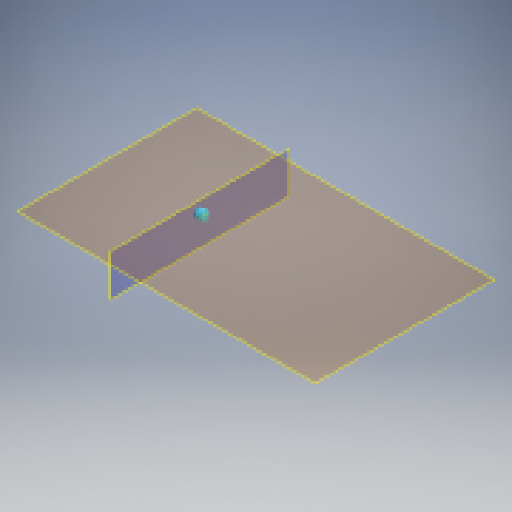
# Autodesk Inventor part: kicker
Saved by Autodesk Inventor 2023 (Build 270158000, 158)
## iProperties
Created: 2025-03-27
Part Number: kicker
Material: Типовые
Document SubType Name: Modeling
Designer: Ivan
Density: 1 g/cm^3
Appearance: Серо-синий
Author: Ivan
Autodesk Inventor part; units mm, degrees
ref_plane "YZ Plane" through (0, 0, 0) normal (1, 0, 0) x (0, 1, 0)
ref_plane "XZ Plane" through (0, 0, 0) normal (0, 1, 0) x (-1, 0, 0)
ref_plane "XY Plane" through (0, 0, 0) normal (0, 0, 1) x (1, 0, 0)
sketch "Эскиз1" plane through (0, 0, 0) normal (1, 0, 0) x (0, 1, 0)
  circle A0 centre (0, 0) radius 2.067 construction
  circle A1 centre (0, 0) radius 5
  circle A2 centre (0, 0) radius 6
  circle A3 centre (0, 0) radius 2.467 projected
  point P0 (0, 0)
  dimension "d1" = 10
  dimension "d2" = 12
  constraints: 2 centre point, 2 coincident
  measures "d1" diameter of A1
  measures "d2" diameter of A2
extrude "Выдавливание1" add sketch "Эскиз1" along normal blind 6.7 contours A2
sketch "Эскиз4" plane through (0, 0, 0) normal (-1, 0, 0) x (0, 0, 1)
  circle A0 centre (0, 0) radius 6 projected
  circle A1 centre (0, 0) radius 5 projected
  point P0 (0, 0)
extrude "Выдавливание2" add sketch "Эскиз4" along normal blind 2.64 contours A0 | A1
ref_plane "РабПлоскость1" through (0, 0, 0) normal (0, 1, 0) x (-1, 0, 0)
sketch "Эскиз5" plane through (0, 0, 0) normal (0, 1, 0) x (-1, 0, 0)
  line L0 (2.64, -6) -> (-6.7, -6) projected
  line L1 (-5, 6) -> (0, 6)
  line L2 (0, 6) -> (0, -6)
  line L3 (0, -6) -> (-5, -6)
  line L4 (-5, -6) -> (-5, 6)
  line L5 (2.64, 6) -> (-6.7, 6) projected
  line L6 (0, 6) -> (0, -6) projected
  point P0 (0, 0)
  dimension "d7" = 5
  constraints: 8 end point, 3 point on line, 2 parallel, 1 horizontal, 1 perpendicular
  measures "d7" distance from line of L1.start L2
extrude "Выдавливание3" cut sketch "Эскиз5" against normal through all
sketch "Эскиз6" plane through (5, 0, 5) normal (-1, 0, 0) x (0, 0, 1)
  circle A0 centre (-5, 0) radius 5 projected
  circle A1 centre (-5, 0) radius 2.467 projected
extrude "Выдавливание4" add sketch "Эскиз6" against normal up to surface (1.7 mm away)
sketch "Эскиз7" plane through (5, 0, 5) normal (-1, 0, 0) x (0, 0, 1)
  line L0 (-1, 0) -> (-1, -2.3094) projected
  line L1 (-9, -2.3094) -> (-9, 0) projected
  circle A0 centre (-5, 0) radius 6 projected
  line L2 (-0.75, -4.2353) -> (-0.75, -2.6339)
  line L3 (1, 0) -> (0, 0) projected
  line L4 (-10, 0) -> (-11, 0) projected
  line L5 (-9.25, -2.6339) -> (-9.25, -4.2353)
  line L6 (-0.75, -2.6339) -> (-0.75, 4.2353)
  line L7 (-9.25, -2.6339) -> (-9.25, 4.2353)
  point P0 (-5, 0)
  point P1 (-9.25, -3.4346)
  dimension "d12" = 0.25
  dimension "d13" = 0.25
  constraints: 8 end point, 4 point on circle, 2 parallel, 2 vertical, 1 midpoint
  measures "d12" distance between parallel lines of L2 L0
  measures "d13" distance from line of point (-9.25, -3.435) L1
extrude "Выдавливание5" add sketch "Эскиз7" along normal up to surface (5 mm away) contours A0 L2 L6 | L7 L5 A0
chamfer "Фаска1" distance 0.4 angle 45 4 edges at (5, -6, 0) (2.5, -4.2353, 4.25) (2.5, -4.2353, -4.25) (0, -6, 0)
ref_plane "РабПлоскость2" through (0, 0, 0) normal (-1, 0, 0) x (0, 0, 1)
ref_plane "РабПлоскость3" through (0, 0, 0) normal (0, 1, 0) x (-1, 0, 0)
sketch "Эскиз9" plane through (0, 0, 0) normal (0, 1, 0) x (-1, 0, 0)
  line L0 (2.64, -6) -> (2.64, 6) projected
  arc A0 (2.64, 6) -> (2.64, -6) centre (47.44, 0) ccw
  line L1 (2.24, 0) -> (2.64, 0)
  point P0 (0, 0)
  dimension "d19" = 0.4
  constraints: 3 point on circle, 2 end point, 1 centre point, 1 midpoint
  measures "d19" distance from line of L1.start L0
revolve "Вращение1" cut sketch "Эскиз9" angle 360 about axis through (-2.24, 0, 0) along (-1, 0, 0) picked at (2.566, 3.3355) contours L1 A0 L0
chamfer "Фаска2" distance 0.1 angle 45 1 edges at (-2.64, 0, -6)
equation "\"d13\" = d12"
